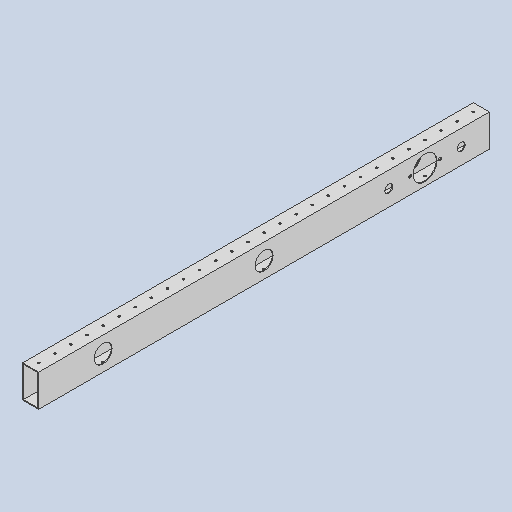
# Autodesk Inventor part: VersaFrame 28in
Saved by Autodesk Inventor 2022 (Build 260153000, 153)
## iProperties
Created: 2020-01-13
Part Number: VersaFrame 28in
Material: Generic
Document SubType Name: Modeling
Designer: aidan
Density: 1 g/cm^3
Appearance: Default
Author: aidan
Autodesk Inventor part; units mm, degrees
ref_plane "YZ Plane" through (0, 0, 0) normal (1, 0, 0) x (0, 1, 0)
ref_plane "XZ Plane" through (0, 0, 0) normal (0, 1, 0) x (-1, 0, 0)
ref_plane "XY Plane" through (0, 0, 0) normal (0, 0, 1) x (1, 0, 0)
sketch "Sketch1" plane through (0, 0, 0) normal (0, 0, 1) x (1, 0, 0)
  line L0 (-12.1708, 16.0073) -> (13.2292, 16.0073)
  line L1 (13.2292, 16.0073) -> (13.2292, -34.7927)
  line L2 (13.2292, -34.7927) -> (-12.1708, -34.7927)
  line L3 (-12.1708, -34.7927) -> (-12.1708, 16.0073)
  line L4 (11.9592, 14.7373) -> (-10.9008, 14.7373)
  line L5 (-10.9008, 14.7373) -> (-10.9008, -33.5227)
  line L6 (-10.9008, -33.5227) -> (11.9592, -33.5227)
  line L7 (11.9592, -33.5227) -> (11.9592, 14.7373)
  point P0 (0, 0)
  dimension "d0" = 25.4
  dimension "d1" = 50.8
  dimension "d2" = 1.27
  constraints: 16 end point, 4 parallel, 2 perpendicular, 1 horizontal, 3 other
  measures "d0" distance of L0.start L0.end
  measures "d1" distance of L0.end L1.end
  measures "d2" distance between parallel lines of L0 L4
extrude "Extrusion1" add sketch "Sketch1" along normal blind 711.2
sketch "Sketch2" plane through (-12.1708, 16.0073, 0) normal (0, 1, 0) x (1, 0, 0)
  circle A0 centre (12.7, -12.7) radius 1.7272
  line L0 (25.4, 0) -> (0, 0) projected
  line L1 (0, 0) -> (0, -711.2) projected
  point P0 (12.1708, 0)
  dimension "d5" = 3.4544
  dimension "d6" = 12.7
  dimension "d7" = 12.7
  constraints: 1 centre point
  measures "d5" diameter of A0
  measures "d6" distance from line of L0 A0.centre
  measures "d7" distance from line of L1 A0.centre
extrude "Extrusion2" cut sketch "Sketch2" against normal through all
pattern_linear "Rectangular Pattern1" count 71 spacing 25.4 along (0, 0, 1) of "Extrusion2"
sketch "Sketch3" plane through (13.2292, -34.7927, 0) normal (1, 0, 0) x (0, 0, -1)
  circle A0 centre (-101.6, 25.4) radius 19.05
  circle A1 centre (-101.6, 25.4) radius 23.8125 construction
  circle A2 centre (-125.4125, 25.4) radius 2.4892
  circle A3 centre (-77.7875, 25.4) radius 2.4892
  line L0 (-406.4, 34.925) -> (-381, 15.875) construction
  line L1 (-711.2, 50.8) -> (-711.2, 0) construction
  line L2 (-711.2, 25.4) -> (0, 25.4) construction
  line L3 (0, 50.8) -> (0, 0) construction
  circle A4 centre (-609.6, 25.4) radius 14.2875
  circle A5 centre (-355.6, 25.4) radius 14.2875
  circle A6 centre (-44.45, 25.4) radius 6.35
  circle A7 centre (-158.75, 25.4) radius 6.35
  line L4 (0, 0) -> (0, 50.8) projected
  point P0 (0, 34.7927)
  point P1 (-393.7, 25.4)
  point P2 (-624.3413, 25.4)
  point P3 (-134.62, 25.4)
  dimension "d15" = 38.1
  dimension "d16" = 47.625
  dimension "d17" = 4.9784
  dimension "d18" = 4.9784
  dimension "d25" = 28.575
  dimension "d27" = 28.575
  dimension "d29" = 12.7
  dimension "d30" = 12.7
  dimension "d31" = 355.6
  dimension "d33" = 101.6
  dimension "d34" = 101.6
  dimension "d35" = 57.15
  dimension "d36" = 57.15
  dimension "d37" = 77.7875
  dimension "d38" = 125.4125
  dimension "d39" = 158.75
  dimension "d40" = 44.45
  constraints: 8 centre point, 6 midpoint, 4 end point, 3 coincident, 3 horizontal alignment, 2 point on circle, 2 point on line
  measures "d15" diameter of A0
  measures "d16" diameter of A1
  measures "d17" diameter of A2
  measures "d18" diameter of A3
  measures "d25" diameter of A4
  measures "d27" diameter of A5
  measures "d29" diameter of A6
  measures "d30" diameter of A7
  measures "d31" distance from line of L1 A5.centre
  measures "d33" distance from line of L1 A4.centre
  measures "d34" distance from line of L3 A0.centre
  measures "d35" distance of A0.centre A6.centre
  measures "d36" distance of A0.centre A7.centre
  measures "d37" distance from line of L3 A3.centre
  measures "d38" distance from line of A2.centre L3
  measures "d39" distance from line of L3 A7.centre
  measures "d40" distance from line of L3 A6.centre
extrude "Extrusion3" cut sketch "Sketch3" against normal through all
equation "\"d3\" = d13"
equation "\"d31\" = 0.5 * d13"
equation "\"d33\" = d32"
equation "\"d34\" = d32"
equation "\"d10\" = d14"
equation "\"d13\" = 711.2"
equation "\"d14\" = d13"
equation "\"d32\" = 101.6"
body "Solid1"
